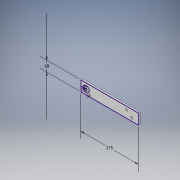
# Autodesk Inventor part: Lagerstuetze_kurz
Saved by Autodesk Inventor 2018 (Build 220112000, 112)
## iProperties
Created: 2018-01-29
Part Number: Lagerstuetze_kurz
Material: Generisch
Document SubType Name: Modeling
Designer: Julian
Density: 1 g/cm^3
Appearance: Vorgabe
Author: Julian
Autodesk Inventor part; units mm, degrees
ref_plane "YZ Plane" through (0, 0, 0) normal (1, 0, 0) x (0, 1, 0)
ref_plane "XZ Plane" through (0, 0, 0) normal (0, 1, 0) x (-1, 0, 0)
ref_plane "XY Plane" through (0, 0, 0) normal (0, 0, 1) x (1, 0, 0)
sketch "Skizze1" plane through (0, 0, 0) normal (0, 1, 0) x (-1, 0, 0)
  line L0 (0, 0) -> (275, 0)
  line L1 (275, 0) -> (275, -50)
  line L2 (275, -50) -> (0, -50)
  line L3 (0, -50) -> (0, 0)
  line L4 (275, 0) -> (275, -25)
  line L5 (275, -25) -> (250, -25)
  circle A0 centre (250, -25) radius 15
  dimension "d0" = 275
  dimension "d1" = 50
  dimension "d2" = 25
  dimension "d3" = 30
  constraints: 12 end point, 2 parallel, 2 perpendicular, 1 centre point, 1 coincident, 1 horizontal, 1 midpoint
  measures "d0" distance of L1.end L2.end
  measures "d1" distance of L0.end L1.end
  measures "d2" distance of L4.end L5.end
  measures "d3" diameter of A0
extrude "Extrusion1" add sketch "Skizze1" along normal blind 9
sketch "Skizze2" plane through (0, 9, 0) normal (0, 1, 0) x (1, 0, 0)
  line L0 (0, 0) -> (0, 50) projected
  line L1 (0, 50) -> (-30, 50)
  line L2 (-30, 50) -> (-30, 35)
  line L3 (0, 0) -> (-55, 0)
  line L4 (-275, 0) -> (0, 0) projected
  line L5 (-55, 0) -> (-70, 0)
  line L6 (-70, 0) -> (-55, 0)
  line L7 (-55, 0) -> (-55, 15)
  dimension "d6" = 30
  dimension "d7" = 15
  dimension "d8" = 55
  dimension "d9" = 15
  dimension "d10" = 15
  constraints: 12 end point, 2 perpendicular, 2 point on line, 1 collinear, 1 horizontal
  measures "d6" distance of L0.end L1.end
  measures "d7" distance of L1.end L2.end
  measures "d8" distance of L0.start L3.end
  measures "d9" distance of L3.end L5.end
  measures "d10" distance of L3.end L7.end
hole "Bohrung1" at (-55, 9, -15) at (-30, 9, -35) direction (0, -1, 0) diameter 10 depth 10 tip angle 118
